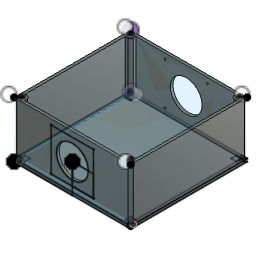
main box v3 (Autodesk Fusion 360 design; units mm, degrees)
Autodesk Fusion 360 part; units mm, degrees
note: some values were not read from the file. Set by a fixed rule: which sketch regions a step uses.
sketch "Sketch1" plane through (0, 0, 0) normal (0, 1, 0) x (1, 0, 0)
  line L0 (0, 0) -> (220, 0)
  line L1 (220, 0) -> (220, -220)
  line L2 (220, -220) -> (0, -220)
  line L3 (0, -220) -> (0, 0)
  dimension "d1" = 220
  dimension "d2" = 220
  constraint horizontal L0
  constraint vertical L1
  constraint horizontal L2
  constraint vertical L3
  constraint coincident L0.start L3.end
  measures "d1" distance of L0.start L0.end
  measures "d2" distance of L0.start L2.end
extrude "Extrude1" add sketch "Sketch1" along normal blind 5
sketch "Sketch2" plane through (0, 5, 0) normal (0, 1, 0) x (-1, 0, 0)
  line L0 (0, 220) -> (-220, 220)
  line L1 (-220, 220) -> (-220, 0)
  line L2 (-220, 0) -> (0, 0)
  line L3 (0, 0) -> (0, 220)
  line L4 (0, 0) -> (-10, 0)
  line L5 (-10, 220) -> (0, 220)
  line L6 (0, 220) -> (0, 0)
  line L7 (0, 0) -> (-5, 0)
  line L8 (-5, 0) -> (-5, 220)
  line L9 (-5, 220) -> (0, 220)
  line L10 (0, 220) -> (0, 0)
  line L11 (0, 0) -> (-220, 0)
  line L12 (-220, 0) -> (-220, 5)
  line L13 (-220, 5) -> (0, 5)
  line L14 (0, 5) -> (0, 0)
  line L15 (0, 220) -> (-220, 220)
  line L16 (-220, 220) -> (-220, 215)
  line L17 (-220, 215) -> (0, 215)
  line L18 (0, 215) -> (0, 220)
  line L19 (-220, 220) -> (-215, 220)
  line L20 (-215, 220) -> (-215, 0)
  line L21 (-215, 0) -> (-220, 0)
  line L22 (-220, 0) -> (-220, 220)
  dimension "d5" = 5
  dimension "d6" = 5
  constraint horizontal L4
  constraint horizontal L5
  constraint vertical L6
  constraint coincident L0 L5.start
  constraint coincident L2.end L3.start
  constraint horizontal L7
  constraint vertical L8
  constraint horizontal L9
  constraint vertical L10
  constraint midpoint L5 L8.end
  constraint horizontal L11
  constraint vertical L12
  constraint horizontal L13
  constraint vertical L14
  constraint horizontal L15
  constraint vertical L16
  constraint horizontal L17
  constraint vertical L18
  constraint coincident L1 L16.end
  constraint coincident L0.start L3.end
  constraint horizontal L19
  constraint vertical L20
  constraint horizontal L21
  constraint vertical L22
  constraint coincident L0.end L1.start
  measures "d5" distance of L2.end L13.end
  measures "d6" distance of L0.end L19.end
extrude "Extrude2" add sketch "Sketch2" along normal blind 100 contours L0 L3 L5 L6 L8 L9 L10 L15 L17 L18 | L0 L5 L8 L15 L17 L20 | L3 L6 L8 L10 L13 L17 | L2 L3 L4 L6 L7 L8 L10 L11 L13 L14 | L0 L1 L15 L16 L17 L19 L20 L22 | L2 L4 L8 L11 L13 L20 | L1 L13 L17 L20 L22 | L1 L2 L11 L12 L13 L20 L21 L22
sketch "Sketch3" plane through (0, 0, 5) normal (0, 0, 1) x (1, 0, 0)
  line L0 (5, 5) -> (215, 5)
  line L1 (215, 5) -> (215, 105)
  line L2 (215, 105) -> (5, 105)
  line L3 (5, 105) -> (5, 5)
sketch "Sketch4" plane through (0, 5, 0) normal (0, 1, 0) x (-1, 0, 0)
  line L0 (-5, 5) -> (-5, 215)
  line L1 (-5, 215) -> (-215, 215)
  line L2 (-215, 215) -> (-215, 5)
  line L3 (-215, 5) -> (-5, 5)
  line L4 (-5, 5) -> (-15, 5)
  line L5 (-15, 5) -> (-15, 15)
  line L6 (-15, 15) -> (-5, 15)
  line L7 (-5, 15) -> (-5, 5)
  line L8 (-215, 5) -> (-205, 5)
  line L9 (-205, 5) -> (-205, 15)
  line L10 (-205, 15) -> (-215, 15)
  line L11 (-215, 15) -> (-215, 5)
  line L12 (-5, 215) -> (-15, 215)
  line L13 (-15, 215) -> (-15, 205)
  line L14 (-15, 205) -> (-5, 205)
  line L15 (-5, 205) -> (-5, 215)
  line L16 (-215, 215) -> (-205, 215)
  line L17 (-205, 215) -> (-205, 205)
  line L18 (-205, 205) -> (-215, 205)
  line L19 (-215, 205) -> (-215, 215)
  dimension "d10" = 10
  dimension "d11" = 10
  dimension "d12" = 10
  dimension "d13" = 10
  dimension "d14" = 10
  dimension "d15" = 10
  dimension "d16" = 10
  dimension "d17" = 10
  constraint horizontal L4
  constraint vertical L5
  constraint horizontal L6
  constraint vertical L7
  constraint coincident L0.start L3.end
  constraint horizontal L8
  constraint vertical L9
  constraint horizontal L10
  constraint vertical L11
  constraint coincident L2.end L3.start
  constraint horizontal L12
  constraint vertical L13
  constraint horizontal L14
  constraint vertical L15
  constraint coincident L0.end L1.start
  constraint horizontal L16
  constraint vertical L17
  constraint horizontal L18
  constraint vertical L19
  constraint coincident L1.end L2.start
  measures "d10" distance of L0.start L4.end
  measures "d11" distance of L0.start L6.end
  measures "d12" distance of L2.end L8.end
  measures "d13" distance of L2.end L10.end
  measures "d14" distance of L0.end L12.end
  measures "d15" distance of L0.end L14.end
  measures "d16" distance of L1.end L16.end
  measures "d17" distance of L1.end L18.end
extrude "Extrude3" add sketch "Sketch4" along normal blind 100 contours L0 L3 L4 L5 L6 L7 | L0 L1 L12 L13 L14 L15 | L2 L3 L8 L9 L10 L11 | L1 L2 L16 L17 L18 L19
fillet "Fillet1" radius 5 4 edges at (205, 55, 15) (15, 55, 15) (15, 55, 205) (205, 55, 205)
sketch "Sketch5" plane through (0, 0, 220) normal (0, 0, 1) x (1, 0, 0)
  line L0 (0, 0) -> (220, 0)
  line L1 (220, 0) -> (220, 105)
  line L2 (220, 105) -> (0, 105)
  line L3 (0, 105) -> (0, 0)
  line L4 (0, 0) -> (110, 0)
  line L5 (110, 0) -> (110, 55)
  line L6 (110, 55) -> (150, 55)
  line L7 (150, 55) -> (150, 15)
  line L8 (150, 15) -> (110, 15)
  line L9 (110, 15) -> (110, 55)
  line L10 (150, 15) -> (70, 15)
  line L11 (70, 15) -> (70, 95)
  line L12 (70, 95) -> (150, 95)
  line L13 (150, 95) -> (150, 15)
  circle A0 centre (110, 55) radius 30
  dimension "d22" = 55
  dimension "d23" = 40
  dimension "d24" = 40
  dimension "d25" = 80
  dimension "d26" = 80
  dimension "d27" = 60
  constraint coincident L0.start L3.end
  constraint midpoint L0 L4.end
  constraint perpendicular L2 L5
  constraint horizontal L6
  constraint vertical L7
  constraint horizontal L8
  constraint vertical L9
  constraint horizontal L10
  constraint vertical L11
  constraint horizontal L12
  constraint vertical L13
  constraint coincident L5.end L6.start
  measures "d22" distance of L4.end L5.end
  measures "d23" distance of L5.end L6.end
  measures "d24" distance of L5.end L8.end
  measures "d25" distance of L7.end L10.end
  measures "d26" distance of L7.end L12.end
  measures "d27" diameter of A0
extrude "Extrude4" cut sketch "Sketch5" against normal blind 270 contours L5 L6 L9 A0 | L5 L6 L9 A0
hole "Hole1" at (70, 95, 220) at (150, 95, 220) at (70, 15, 220) at (150, 15, 220) direction (0, 0, -1) diameter 3.5 depth 10000 tip angle 118
sketch "Sketch6" plane through (0, 105, 0) normal (0, 1, 0) x (-1, 0, 0)
  arc A0 (-210, 205) -> (-205, 210) centre (-210, 210) ccw
  line L0 (-205, 210) -> (-205, 215)
  line L1 (-205, 215) -> (-15, 215)
  line L2 (-15, 215) -> (-15, 210)
  arc A1 (-15, 210) -> (-10, 205) centre (-10, 210) ccw
  line L3 (-10, 205) -> (-5, 205)
  line L4 (-5, 205) -> (-5, 15)
  line L5 (-5, 15) -> (-10, 15)
  arc A2 (-10, 15) -> (-15, 10) centre (-10, 10) ccw
  line L6 (-15, 10) -> (-15, 5)
  line L7 (-15, 5) -> (-205, 5)
  line L8 (-205, 5) -> (-205, 10)
  arc A3 (-205, 10) -> (-210, 15) centre (-210, 10) ccw
  line L9 (-210, 15) -> (-215, 15)
  line L10 (-215, 15) -> (-215, 205)
  line L11 (-215, 205) -> (-210, 205)
  line L12 (0, 0) -> (0, 220)
  line L13 (0, 220) -> (-220, 220)
  line L14 (-220, 220) -> (-220, 0)
  line L15 (-220, 0) -> (0, 0)
  line L16 (0, 0) -> (-7.0711, 7.0711)
  line L17 (0, 0) -> (10, 0) construction
  line L18 (-220, 0) -> (-212.9289, 7.0711)
  line L19 (-220, 0) -> (-210, 0) construction
  line L20 (0, 220) -> (-7.0711, 212.9289)
  line L21 (0, 220) -> (10, 220) construction
  line L22 (-220, 220) -> (-212.9289, 212.9289)
  line L23 (-220, 220) -> (-210, 220) construction
  dimension "d33" = 135
  dimension "d34" = 10
  dimension "d35" = 45
  dimension "d36" = 10
  dimension "d37" = 135
  dimension "d38" = 10
  dimension "d39" = 10
  dimension "d40" = 45
  constraint horizontal L17
  constraint coincident L12.start L15.end
  constraint horizontal L19
  constraint coincident L14.end L15.start
  constraint horizontal L21
  constraint coincident L12.end L13.start
  constraint horizontal L23
  constraint coincident L13.end L14.start
  measures "d33" angle of L16 L17
  measures "d34" distance of L12.start L16.end
  measures "d35" angle of L18 L19
  measures "d36" distance of L14.end L18.end
  measures "d37" angle of L20 L21
  measures "d38" distance of L12.end L20.end
  measures "d39" distance of L13.end L22.end
  measures "d40" angle of L22 L23
hole "Hole2" at (7.0711, 105, 212.9289) at (212.9289, 105, 212.9289) at (212.9289, 105, 7.0711) at (7.0711, 105, 7.0711) direction (0, -1, 0) diameter 4.7 depth 4.3 tip angle 180
hole "Hole3" at (7.0711, 105, 212.9289) at (212.9289, 105, 212.9289) at (212.9289, 105, 7.0711) at (7.0711, 105, 7.0711) direction (0, -1, 0) diameter 3.5 depth 8 tip angle 180
fillet "Fillet2" radius 5 4 edges at (220, 52.5, 220) (0, 52.5, 220) (0, 52.5, 0) (220, 52.5, 0)
